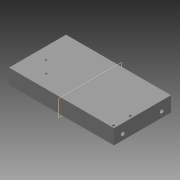
# Autodesk Inventor part: tapa
Saved by Autodesk Inventor 2015 (Build 190159000, 159)
## iProperties
Created: 2015-02-18
Part Number: tapa
Material: Genérico
Document SubType Name: Modeling
Designer: jorge
Density: 1 g/cm^3
Appearance: Valor por defecto
Author: jorge
Autodesk Inventor part; units mm, degrees
ref_plane "YZ Plane" through (0, 0, 0) normal (1, 0, 0) x (0, 1, 0)
ref_plane "XZ Plane" through (0, 0, 0) normal (0, 1, 0) x (-1, 0, 0)
ref_plane "XY Plane" through (0, 0, 0) normal (0, 0, 1) x (1, 0, 0)
sketch "Boceto1" plane through (0, 0, 0) normal (0, 0, 1) x (1, 0, 0)
  line L0 (-116.5, 26.5) -> (-116.5, -26.5) projected
  line L1 (-1.5, 26.5) -> (-1.5, -26.5) projected
  line L2 (-116.5, -26.5) -> (-1.5, -26.5)
  line L3 (-1.5, -26.5) -> (-1.5, 26.5)
  line L4 (-1.5, 26.5) -> (-116.5, 26.5)
  line L5 (-116.5, 26.5) -> (-116.5, -26.5)
  point P0 (0, 0)
  constraints: 8 end point, 2 parallel, 1 horizontal, 1 perpendicular
extrude "interior" add sketch "Boceto1" against normal blind 3
sketch "Boceto2" plane through (0, 0, 0) normal (0, 0, 1) x (1, 0, 0)
  line L0 (-119.5, -31.5) -> (-119.5, 31.5) projected
  line L1 (1.5, -31.5) -> (1.5, 31.5) projected
  line L2 (-119.5, -31.5) -> (1.5, -31.5)
  line L3 (1.5, -31.5) -> (1.5, 31.5)
  line L4 (1.5, 31.5) -> (-119.5, 31.5)
  line L5 (-119.5, 31.5) -> (-119.5, -31.5)
  point P0 (0, 0)
  constraints: 8 end point, 2 parallel, 1 horizontal, 1 perpendicular
extrude "superior" add sketch "Boceto2" along normal blind 3
sketch "Boceto3" plane through (0, 0, 3) normal (0, 0, 1) x (1, 0, 0)
  line L0 (-119.5, -31.5) -> (1.5, -31.5)
  line L1 (1.5, -31.5) -> (1.5, 31.5)
  line L2 (1.5, 31.5) -> (-119.5, 31.5)
  line L3 (-119.5, 31.5) -> (-119.5, -31.5)
  line L4 (-122.5, 34.5) -> (4.5, 34.5)
  line L5 (4.5, 34.5) -> (4.5, -34.5)
  line L6 (4.5, -34.5) -> (-122.5, -34.5)
  line L7 (-122.5, -34.5) -> (-122.5, 34.5)
  point P0 (0, 0)
  dimension "d4" = 3
  constraints: 16 end point, 4 parallel, 2 perpendicular, 1 horizontal, 3 other
  measures "d4" distance between parallel lines of L2 L4
extrude "laterales" add sketch "Boceto3" against normal blind 18
sketch "Boceto4" plane through (4.5, -34.5, 3) normal (1, 0, 0) x (0, 0, -1)
  circle A0 centre (11.0023, 11) radius 3 projected
  circle A1 centre (11.0023, 58) radius 2.5 projected
  point P0 (3, 34.5)
hole "Agujero1" at (4.5, -23.5, -8.0023) at (4.5, 23.5, -8.0023) direction (-1, 0, 0) diameter 5 depth 3
ref_plane "Plano de trabajo1" through (-59, -34.5, 3) normal (1, 0, 0) x (0, 0, -1)
mirror "Simetría1" about plane through (-59, -34.5, 3) normal (1, 0, 0) of "Agujero1"
sketch "Boceto5" plane through (0, 0, 3) normal (0, 0, 1) x (1, 0, 0)
  circle A0 centre (1.5, -32) radius 1.25 projected
  circle A1 centre (1.5, -11.7293) radius 1.25 projected
  point P0 (0, 0)
hole "Agujero2" at (1.5, -11.7293, 3) at (1.5, -32, 3) direction (0, 0, -1) diameter 2.5 depth 5 tip angle 118
sketch "Boceto6" plane through (0, 0, 3) normal (0, 0, 1) x (1, 0, 0)
  circle A0 centre (-108.0086, -4.2586) radius 1 projected
  circle A1 centre (-93.4586, -18.4086) radius 1 projected
  point P0 (0, 0)
hole "Agujero3" at (-108.0086, -4.2586, 3) at (-93.4586, -18.4086, 3) direction (0, 0, -1) diameter 2 depth 5 tip angle 118
fillet "Empalme1" radius 2 7 edges at (-116.5, -26.5, -1.5) (-116.5, 26.5, -1.5) (-1.5, 26.5, -1.5) (-1.5, -26.5, -1.5) (1.5, 31.5, -7.5) (-119.5, -31.5, -7.5) (-119.5, 31.5, -7.5)
